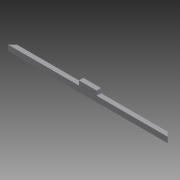
# Autodesk Inventor part: Rail
Saved by Autodesk Inventor 2011 (Build 150239000, 239)
## iProperties
Created: 2014-08-04
Part Number: Rail
Material: Por defecto
Document SubType Name: Chapa
Designer: amatiasq
Density: 1 g/cm^3
Sheet Metal Rule: Por defecto_mm
Author: amatiasq
Autodesk Inventor part; units mm, degrees
ref_plane "YZ Plane" through (0, 0, 0) normal (1, 0, 0) x (0, 1, 0)
ref_plane "XZ Plane" through (0, 0, 0) normal (0, 1, 0) x (-1, 0, 0)
ref_plane "XY Plane" through (0, 0, 0) normal (0, 0, 1) x (1, 0, 0)
sketch "Boceto1" plane through (0, 0, 0) normal (0, 0, 1) x (1, 0, 0)
  line L0 (0, 0) -> (72, 0)
  line L1 (2, 2) -> (0, 0)
  line L2 (2, 2) -> (70, 2)
  line L3 (70, 2) -> (72, 0)
  dimension "d0" = 72
  dimension "d1" = 68
  constraints: 8 end point, 1 horizontal, 1 parallel, 1 perpendicular
  measures "d0" distance of L0.start L0.end
  measures "d1" distance of L1.start L2.end
extrude "Extrusión1" add sketch "Boceto1" along normal blind 2.5
sketch "Boceto2" plane through (0, 0, 2.5) normal (0, 0, 1) x (1, 0, 0)
  line L0 (72, 0) -> (0, 0) projected
  line L1 (2, 2) -> (70, 2) projected
  line L2 (32, 0) -> (40, 0)
  line L3 (40, 0) -> (40, 2)
  line L4 (40, 2) -> (32, 2)
  line L5 (32, 2) -> (32, 0)
  dimension "d4" = 8
  constraints: 8 end point, 2 parallel, 2 point on line, 1 horizontal, 1 perpendicular
  measures "d4" distance of L4.end L3.end
extrude "Extrusión2" add sketch "Boceto2" along normal blind 2
equation "\"Radio_pliegue\" = Grosor"
equation "\"Anchura_desahogo_plegado\" = Grosor"
equation "\"Profundidad_desahogo_plegado\" = 0.5 * Grosor"
equation "\"Tamaño_destalonado\" = 4 * Grosor"
equation "\"Remanente_mínimo\" = 2 * Grosor"
equation "\"Radiodetransición\" = Radio_pliegue"
equation "\"Tamaño_de_radio_de_Jacobi\" = Radio_pliegue"
equation "\"TamañoSeparación\" = Grosor"
equation "\"Grosor\" = 0.5"
